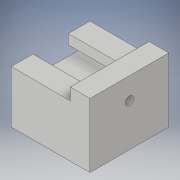
# Autodesk Inventor part: tenshoner base
Saved by Autodesk Inventor 2019 (Build 230136000, 136)
## iProperties
Created: 2019-12-07
Part Number: tenshoner base
Material: Generic
Document SubType Name: Modeling
Designer: User
Density: 1 g/cm^3
Appearance: Default
Author: User
Autodesk Inventor part; units mm, degrees
ref_plane "YZ Plane" through (0, 0, 0) normal (1, 0, 0) x (0, 1, 0)
ref_plane "XZ Plane" through (0, 0, 0) normal (0, 1, 0) x (-1, 0, 0)
ref_plane "XY Plane" through (0, 0, 0) normal (0, 0, 1) x (1, 0, 0)
sketch "Sketch1" plane through (0, 0, 0) normal (1, 0, 0) x (0, 1, 0)
  line L0 (0, 0) -> (16.891, 0)
  line L1 (16.891, 0) -> (16.891, -25.4)
  line L2 (16.891, -25.4) -> (0, -25.4)
  line L3 (0, -25.4) -> (0, 0)
  line L4 (16.891, -6.985) -> (13.716, -6.985)
  line L5 (13.716, -6.985) -> (13.716, -3.175)
  line L6 (13.716, -3.175) -> (10.541, -3.175)
  line L7 (10.541, -3.175) -> (10.541, -22.225)
  line L8 (10.541, -22.225) -> (13.716, -22.225)
  line L9 (13.716, -22.225) -> (13.716, -18.415)
  line L10 (13.716, -18.415) -> (16.891, -18.415)
  dimension "d0" = 25.4
  dimension "d1" = 11.43
  dimension "d2" = 19.05
  dimension "d3" = 3.81
  dimension "d4" = 6.985
  dimension "d5" = 3.175
  dimension "d6" = 6.35
  dimension "d7" = 16.891
  constraints: 22 end point, 6 perpendicular, 4 point on line, 2 horizontal, 2 parallel
  measures "d0" distance of L0.end L1.end
  measures "d1" distance between parallel lines of L4 L10
  measures "d2" distance between parallel lines of L8 L6
  measures "d3" distance between parallel lines of L4 L6
  measures "d4" distance between parallel lines of L0 L4
  measures "d5" distance between parallel lines of L7 L5
  measures "d6" distance between parallel lines of L1 L7
  measures "d7" distance between parallel lines of L3 L1
extrude "Extrusion1" add sketch "Sketch1" along normal blind 19.05 contours L0 L1 L4 L5 L6 L7 L8 L9 L10 L2 L3
sketch "Sketch2" plane through (19.05, 0, 0) normal (1, 0, 0) x (0, 0, -1)
  line L0 (0, 0) -> (25.4, 0)
  line L1 (25.4, 0) -> (25.4, 20.701)
  line L2 (25.4, 20.701) -> (0, 20.701)
  line L3 (0, 20.701) -> (0, 0)
  line L4 (25.4, 16.891) -> (18.415, 16.891) projected
  dimension "d10" = 3.81
  dimension "d11" = 25.4
  constraints: 8 end point, 2 parallel, 1 coincident, 1 horizontal, 1 perpendicular
  measures "d10" distance between parallel lines of L2 L4
  measures "d11" distance between parallel lines of L3 L1
extrude "Extrusion2" add sketch "Sketch2" along normal blind 6.35
sketch "Sketch4" plane through (19.05, 0, 0) normal (-1, 0, 0) x (0, 0, 1)
  circle A0 centre (-12.7, 13.716) radius 1.3208
  line L0 (0, 16.891) -> (0, 0) projected
  line L1 (-22.225, 10.541) -> (-3.175, 10.541) projected
  line L2 (-3.175, 13.716) -> (-6.985, 13.716) projected
  dimension "d21" = 2.6416
  dimension "d22" = 12.7
  dimension "d23" = 3.175
  dimension "d24" = 0
  constraints: 1 centre point
  measures "d21" diameter of A0
  measures "d22" distance from line of L0 A0.centre
  measures "d23" distance between parallel lines of L1 L2
  measures "d24" distance from line of L2 A0.centre
extrude "Extrusion3" cut sketch "Sketch4" against normal through all
equation "\"d3\" = -0.5 * d1 + 0.5 * d2"
equation "\"d4\" = -0.5 * d1 + 0.5 * d0"
body "Solid1"
